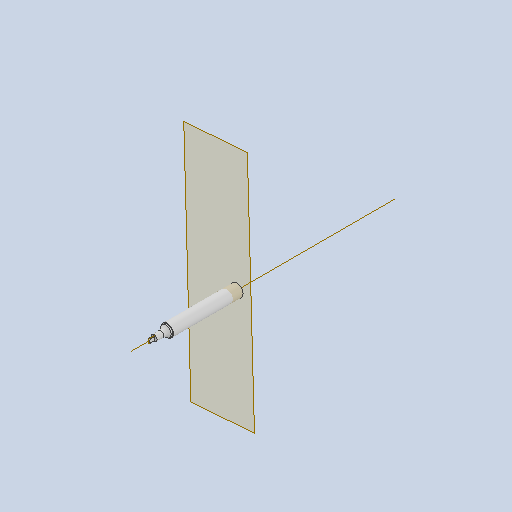
# Autodesk Inventor part: Pelikan426
Saved by Autodesk Inventor 2023.1 (Build 271208000, 208)
## iProperties
Created: 2022-08-29
Part Number: Pelikan426
Material: Generic
Document SubType Name: Modeling
Designer: Daniel Peña
Density: 1 g/cm^3
Appearance: Default
Author: Daniel Peña
Autodesk Inventor part; units mm, degrees
ref_plane "YZ Plane" through (0, 0, 0) normal (1, 0, 0) x (0, 1, 0)
ref_plane "XZ Plane" through (0, 0, 0) normal (0, 1, 0) x (-1, 0, 0)
ref_plane "XY Plane" through (0, 0, 0) normal (0, 0, 1) x (1, 0, 0)
sketch "Sketch1" plane through (0, 0, 0) normal (0, 1, 0) x (-1, 0, 0)
  line L0 (8.2989, 56.0172) -> (16.6489, 56.0172)
  line L1 (16.6489, 56.0172) -> (16.6489, 151.0172)
  line L2 (8.2989, 169.0172) -> (8.2989, 56.0172)
  line L3 (16.6489, 151.0172) -> (15.4989, 151.0172)
  line L4 (15.4989, 151.0172) -> (15.4989, 153.0172)
  line L5 (15.4989, 153.0172) -> (12.2989, 153.0172)
  arc A0 (12.2989, 160.0172) -> (15.4989, 153.0172) centre (21.5551, 160.0172) ccw
  line L6 (12.2989, 160.0172) -> (12.2989, 169.0172)
  line L7 (12.2989, 169.0172) -> (8.2989, 169.0172)
  point P0 (0, 0)
  dimension "d0" = 95
  dimension "d1" = 16.7
  dimension "d2" = 2
  dimension "d3" = 14.4
  dimension "d4" = 7
  dimension "d6" = 8
  dimension "d7" = 18
  constraints: 16 end point, 3 horizontal, 3 perpendicular, 2 point on circle, 1 centre point, 1 parallel, 1 vertical
  measures "d0" distance of L0.end L1.end
  measures "d1" diameter of L1 L2
  measures "d2" distance of L3.end L4.end
  measures "d3" diameter of L4 L2
  measures "d4" distance of L5.end L6.start
  measures "d6" diameter of L6 L2
  measures "d7" distance between parallel lines of L3 L7
revolve "Revolution1" add sketch "Sketch1" angle 360 about axis through (-8.2989, 0, 169.0172) along (0, 0, -1)
ref_plane "Work Plane1" through (-9.719, 47.979, 70.3641) normal (0.0432, 0.0013, 0.9991) x (-0.9986, -0.0296, 0.0432)
ref_plane "Work Plane2" through (-8.2984, 20.4607, -9.4915) normal (1, 0, 0) x (0, 0, -1)
sketch "Sketch3" plane through (-8.2984, 20.4607, -9.4915) normal (1, 0, 0) x (0, 0, -1)
  line L0 (-184.5087, -22.9607) -> (-178.5087, -22.9607) projected
  line L1 (-178.5087, -22.9607) -> (-178.5087, -17.9607) projected
  line L2 (-178.5087, -17.9607) -> (-184.5087, -17.9607) projected
  line L3 (-184.5087, -17.9607) -> (-185.5087, -19.9607) projected
  line L4 (-185.5087, -19.9607) -> (-184.5087, -22.9607) projected
  point P0 (-9.4915, -20.4607)
extrude "Extrusion2" add sketch "Sketch3" along normal mid plane 2
body "Solid1"
